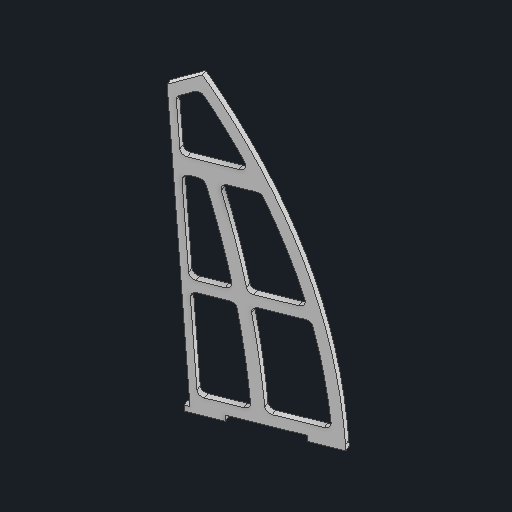
# Autodesk Inventor part: sponson_spanner_bottom
Saved by Autodesk Inventor 2023 (Build 270158030, 158C)
## iProperties
Created: 2022-03-22
Part Number: sponson_spanner_bottom
Material: Generic
Document SubType Name: Modeling
Designer: kardo
Density: 1 g/cm^3
Appearance: Default
Mass: 2.79206 g
Surface Area: 40.129 cm^2
Volume: 2.79206 cm^3
Author: kardo
Autodesk Inventor part; units mm, degrees
ref_plane "YZ Plane" through (0, 0, 0) normal (1, 0, 0) x (0, 1, 0)
ref_plane "XZ Plane" through (0, 0, 0) normal (0, 1, 0) x (-1, 0, 0)
ref_plane "XY Plane" through (0, 0, 0) normal (0, 0, 1) x (1, 0, 0)
derived "parameters_frame.ipt"
derived "stencil_frame.ipt"
sketch "sk_joint_locations" plane through (81.12, 0, 0) normal (1, 0, 0) x (0, 1, 0)
  line L0 (0, 0) -> (122.4, 9.6331) construction
  line L1 (36.465, 28.832) -> (112.2, 28.832) construction
  arc A0 (36.465, 28.832) -> (11.22, 28.376) centre (36.465, -670.197) ccw construction
  line L2 (-241.5001, 19.2432) -> (11.22, 28.376) construction
  line L3 (-345, 16.32) -> (-262.2001, 18.586) construction
  arc A1 (-262.2001, 18.586) -> (-241.5001, 19.2432) centre (-326.8578, 2381.2399) ccw construction
  line L4 (-122.4795, 3121.122) -> (270.8781, -1876.9598) construction
  line L5 (-230.0001, 3089.1136) -> (-230.0001, -1866.0023) construction
  line L6 (-114.9999, 3089.1136) -> (-114.9999, -1866.0023) construction
  line L7 (-345, 3089.1136) -> (-345, -1866.0023) construction
  line L8 (0, 3089.1136) -> (0, -1866.0023) construction
  line L9 (529.622, 47.2379) -> (-602.608, 2.7525) construction
  line L10 (-673.1615, -36.5999) -> (647.9226, 67.3717) construction
  line L11 (193.439, 30.0262) -> (193.1249, 38.02) construction
  line L12 (201.1327, 36.2333) -> (201.7624, 28.2333) construction
  line L13 (0, 14.144) -> (121.9006, 15.9783) construction
  line L14 (-230.0001, 45.8224) -> (-230.0001, 19.6588) construction
  line L15 (-345, 37.3935) -> (-345, 16.32) construction
  line L16 (-114.9999, 50.9907) -> (-114.9999, 23.8147) construction
  line L17 (0, 52.89) -> (0, 27.9705) construction
  line L18 (119.1768, 50.5875) -> (119.7216, 43.6656) construction
  line L19 (120.2663, 36.7438) -> (119.7216, 43.6656) construction
  line L20 (120.2663, 36.7438) -> (120.8111, 29.822) construction
  line L21 (120.8111, 29.822) -> (121.3559, 22.9001) construction
  line L22 (121.3559, 22.9001) -> (121.9006, 15.9783) construction
  line L23 (0, 14.144) -> (0, 0) construction
  line L24 (112.2, 37.536) -> (112.2, 28.832) construction
  line L25 (112.2, 35.548) -> (112.2, 30.82) construction
  spline S0 degree 4 poles (-345, 37.3935) (-258.8686, 45.1235) (-172.5923, 49.7074) (-86.3167, 52.89) (0, 52.89) knots 0 0 0 0 0 1 1 1 1 1
  spline S1 degree 3 poles (0, 52.89) (92.8353, 52.89) (195.0311, 49.5089) (255, 36.448) knots 0 0 0 0 1 1 1 1
  spline S2 degree 2 poles (122.4, 9.6331) (190.08, 14.9596) (255, 36.448) knots 0 0 0 1 1 1
  point P0 (-122.4795, 3121.122)
  point P1 (270.8781, -1876.9598)
  point P2 (193.282, 34.0231)
  point P3 (201.4475, 32.2333)
  point P4 (134.9575, 11.3411)
  point P5 (-345, 26.8568)
  point P6 (-230.0001, 32.7406)
  point P7 (-114.9999, 37.4027)
  point P8 (0, 40.4303)
  point P9 (112.2, 33.184)
sketch "sk_spanner_joints_locations" plane through (0, 122.4, 9.6331) normal (0, 0.9969173, 0.0784591) x (-1, 0, 0)
  line L0 (328.7115, -3.4565) -> (-466.2934, 45.1587) construction
  line L1 (-867.9776, -269.6459) -> (1175.5999, 473.0692) construction
  line L2 (-83.4141, 21.7453) -> (-82.5545, 15.8072) construction
  line L3 (-83.4141, 21.7453) -> (-68.6928, 20.8451) construction
  line L4 (-82.5545, 15.8072) -> (-68.6928, 20.8451) construction
  point P0 (0, 0)
  point P1 (-126.048, 0)
  point P2 (-156, 26.184)
  point P3 (-141.4828, 25.2963)
  point P4 (-97.9313, 22.6331)
  point P5 (-93.4279, 11.8554)
  point P6 (-115.1746, 3.9518)
ref_plane "plane_strnger_outer" through (84.12, 0, 0) normal (1, 0, 0) x (0, 1, 0)
sketch "sk_corner_offset" plane through (0, 122.4, 9.6331) normal (0, 0.9969173, 0.0784591) x (-1, 0, 0)
  line L0 (-156, 26.184) -> (-126.048, 0) construction
  line L1 (-126.048, 0) -> (-81.12, 0) construction
  point P0 (0, 0)
  point P1 (-125.5974, 1.2)
  dimension "d7" = 1.2
  dimension "d8" = 1.2
  constraints: 4 end point, 1 horizontal
  measures "d7" distance from line of L0 point (-125.597, 1.2)
  measures "d8" distance from line of point (-125.597, 1.2) L1
sketch "sk_tip_offset" plane through (81.12, 0, 0) normal (1, 0, 0) x (0, 1, 0)
  spline S0 degree 3 poles (0, 52.89) (92.8353, 52.89) (195.0311, 49.5089) (255, 36.448) knots 0 0 0 0 1 1 1 1 construction
  spline S1 degree 2 poles (122.4, 9.6331) (190.08, 14.9596) (255, 36.448) knots 0 0 0 1 1 1 construction
  spline S2 degree 5 poles (0, 51.69) (14.1108, 51.69) (28.2217, 51.6249) (42.3321, 51.4877) (70.2924, 51.0558) (98.2445, 50.2552) (112.0882, 49.7555) (138.5614, 48.5709) (165.0044, 46.8436) (177.6143, 45.8726) (199.7992, 43.8515) (221.9015, 41.0762) (231.4314, 39.7015) (240.9325, 38.1149) (250.3665, 36.1966) knots 0 0 0 0 0 0 0.280891 0.280891 0.280891 0.556633 0.556633 0.556633 0.808364 0.808364 0.808364 1 1 1 1 1 1
  spline S3 degree 4 poles (122.3058, 10.8294) (154.9158, 13.3957) (187.3327, 18.4882) (219.233, 26.1601) (250.3665, 36.1967) knots 0 0 0 0 0 1 1 1 1 1
  point P0 (0, 0)
  dimension "d9" = 1.2
  dimension "d10" = 1.2
  constraints: 1 coincident, 6 other
sketch "sk_spanner_bottom_base" plane through (126.048, 0, 0) normal (0.341579, -0.07374, 0.9369558) x (-0.1718217, 0.9752166, 0.139391)
  spline S0 degree 2 poles (120.7093, -22.4461) (192.8116, -35.8536) (261.4804, 0) knots 0 0 0 1 1 1 construction
  line L0 (-554.724, 148.5277) -> (631.772, -72.103) projected
  line L1 (120.8616, -21.6267) -> (118.8953, -21.2611)
  line L2 (118.8953, -21.2611) -> (120.858, -10.7062)
  line L3 (120.858, -10.7062) -> (122.8243, -11.0718)
  line L4 (122.8243, -11.0718) -> (127.0545, 11.6767)
  line L5 (127.0545, 11.6767) -> (125.0882, 12.0423)
  line L6 (125.0882, 12.0423) -> (127.2032, 23.4166)
  line L7 (127.2032, 23.4166) -> (129.1695, 23.0509)
  line L8 (129.1695, 23.0509) -> (128.865, 21.4133)
  line L9 (120.7093, -22.4461) -> (0, 0) construction
  spline S1 degree 2 poles (120.8616, -21.6267) (190.6868, -34.6108) (256.9266, 0.886) knots 0 0 0 1 1 1
  point P0 (21.6578, 116.4701)
  point P1 (120.7093, -22.4461)
  point P2 (208.6676, 9.8206)
  point P3 (256.8119, -2.3786)
  point P4 (0, 0)
  point P5 (252.289, -1.5376)
  dimension "d4" = 2
  constraints: 16 end point, 3 parallel, 2 collinear, 2 perpendicular, 1 point on line, 5 other
  measures "d4" distance between parallel lines of L6 L4
extrude "thicken" add sketch "sk_spanner_bottom_base" along normal blind 2
sketch "sk_cut_weight" plane through (126.048, 0, 0) normal (0.341579, -0.07374, 0.9369558) x (-0.1718217, 0.9752166, 0.139391)
  spline S0 degree 2 poles (120.8616, -21.6267) (190.6868, -34.6108) (256.9266, 0.886) knots 0 0 0 1 1 1 construction
  line L0 (-554.724, 148.5277) -> (631.772, -72.103) projected
  line L1 (122.8243, -11.0718) -> (127.0545, 11.6767) construction
  line L2 (129.1695, 23.0509) -> (128.865, 21.4133) projected
  line L3 (208.6676, 9.8206) -> (203.1592, -19.8025) construction
  line L4 (129.1695, 23.0509) -> (204.456, 9.0513)
  line L5 (204.456, 9.0513) -> (204.1515, 7.4137)
  line L6 (210.0504, 6.3168) -> (210.3549, 7.9544)
  line L7 (210.3549, 7.9544) -> (252.5935, 0.1001)
  line L8 (132.3708, 18.3871) -> (203.7247, 5.1187)
  line L9 (203.7247, 5.1187) -> (202.5596, -1.1473)
  line L10 (132.3708, 18.3871) -> (129.6075, 3.5268)
  line L11 (209.6236, 4.0218) -> (206.0153, -15.3831)
  line L12 (252.5935, 0.1001) -> (252.289, -1.5376)
  spline S1 degree 2 poles (124.9394, 0.3024) (164.9691, -7.1411) (205.9134, -4.9909) knots 0 0 0 1 1 1
  line L13 (209.6236, 4.0218) -> (242.7978, -2.147)
  line L14 (201.8092, -5.1825) -> (199.6278, -16.9136)
  line L15 (128.8762, -0.406) -> (125.4604, -18.7756)
  line L16 (170.0141, 11.3873) -> (167.7307, -0.8921)
  line L17 (166.0815, 12.1185) -> (163.7104, -0.6324)
  line L18 (166.9937, -4.8554) -> (163.9159, -21.4073)
  line L19 (162.9745, -4.5901) -> (159.832, -21.4898)
  line L20 (168.0478, 11.7529) -> (161.8719, -21.4595) construction
  line L21 (231.4742, 4.0272) -> (245.7915, -36.4796)
  line L22 (228.4725, 0.5168) -> (231.1826, -7.1508)
  line L23 (252.5935, 0.1001) -> (245.7915, -36.4796)
  spline S2 degree 5 poles (125.4604, -18.7756) (138.0935, -20.8759) (150.8878, -22.0045) (163.7589, -22.0658) (187.8356, -20.1071) (211.2999, -14.4431) (222.0705, -11.0146) (232.5774, -6.8893) (242.7978, -2.147) knots 0 0 0 0 0 0 0.531973 0.531973 0.531973 1 1 1 1 1 1
  spline S3 degree 4 poles (125.6707, 4.235) (135.1013, 2.4813) (144.5985, 1.0809) (154.1417, 0.043) (163.7104, -0.6324) knots 0 0 0 0 0 1 1 1 1 1
  spline S4 degree 4 poles (163.7104, -0.6324) (173.4046, -1.3166) (183.1251, -1.6289) (192.8505, -1.5691) (202.5596, -1.1473) knots 0 0 0 0 0 1 1 1 1 1
  point P0 (21.6578, 116.4701)
  point P1 (167.7307, -0.8921)
  point P2 (128.7343, 3.0587)
  point P3 (139.2857, 19.818)
  dimension "d11" = 3.6057
  dimension "d17" = 4
  dimension "d12" = 2
  dimension "d13" = 4
  dimension "d14" = 4
  dimension "d18" = 4
  dimension "d22" = 60
  dimension "d23" = 4
  dimension "d24" = 4
  constraints: 43 end point, 9 collinear, 7 point on line, 6 parallel, 5 perpendicular, 4 midpoint, 29 other
  measures "d12" distance between parallel lines of L6 L3
  measures "d13" distance between parallel lines of L3 L5
  measures "d14" distance between parallel lines of L4 L8
  measures "d18" distance between parallel lines of L17 L16
  measures "d22" angle of L7 L21
  measures "d23" distance between parallel lines of L22 L21
  measures "d24" distance between parallel lines of L1 L10
extrude "cut_weight" cut sketch "sk_cut_weight" along normal through all both and the other way through all contours L21 L7 L12 L0 | L0 L23 L21 S2 L13 | L13 S2 L21 | L22 S2 L11 L13 | L8 L17 S3 L10 | L8 L9 S4 L16 | S1 L19 S2 L15 | S1 L14 S2 L18
fillet "rounding" radius 2 20 edges at (86.6555, 203.5157, 31.4454) (86.6555, 163.3514, 28.2844) (102.1828, 163.7942, 22.6585) (104.621, 125.6932, 18.771) (86.6555, 125.1809, 25.2803) (86.6555, 159.3637, 27.9705) (102.6283, 159.8192, 22.1833) (86.6555, 197.5342, 30.9746) (96.503, 197.815, 27.4067) (92.6456, 197.7051, 28.8043) (107.7175, 198.1348, 23.3434) (118.7838, 160.2799, 16.3298) (98.8449, 159.7113, 23.5541) (105.2059, 204.0447, 24.7242) (118.0059, 164.2454, 16.9255) (122.1817, 126.1939, 12.4085) (98.3941, 163.6861, 24.0313) (100.8614, 125.586, 20.1332) (86.6555, 222.6286, 32.9496) (93.2748, 226.871, 30.8703)
equation "\"d7\" = shell_thickness"
equation "\"d8\" = shell_thickness"
equation "\"d9\" = shell_thickness"
equation "\"d10\" = shell_thickness"
equation "\"d4\" = bulkhead_thickness"
equation "\"d5\" = bulkhead_thickness"
equation "\"d17\" = bulkhead_inset"
equation "\"d12\" = bulkhead_thickness"
equation "\"d13\" = 2 * bulkhead_thickness"
equation "\"d14\" = bulkhead_inset"
equation "\"d18\" = bulkhead_inset"
equation "\"d23\" = bulkhead_inset"
equation "\"d21\" = 0.5 * bulkhead_inset"
equation "\"d3\" = stringer_thickness"
equation "\"shell_thickness\" = 1.2"
equation "\"bulkhead_thickness\" = 2"
equation "\"bulkhead_inset\" = 4"
equation "\"stringer_thickness\" = 3"
body "Solid1"
